Autodesk Fusion 360 part; units mm, degrees
note: some values were not read from the file. Chosen so that the rebuilt part matches the saved one: where a step ends; which bodies a step acts on; which face or edge a step refers to. Set by a fixed rule: which sketch regions a step uses.
(part 5 of 5)
  spline S19 degree 5 poles (-12.661362, 8.043004) (-12.659845, 8.039125) (-12.656809, 8.031374) (-12.652245, 8.019765) (-12.646142, 8.004321) (-12.638485, 7.985073) (-12.630798, 7.965883) (-12.623082, 7.946751) (-12.615336, 7.927676) (-12.607562, 7.90866) (-12.599758, 7.889701) (-12.591926, 7.8708) (-12.584066, 7.851958) (-12.576177, 7.833174) (-12.568261, 7.814449) (-12.560317, 7.795783) (-12.552346, 7.777176) (-12.544347, 7.758628) (-12.536322, 7.74014) (-12.52827, 7.721712) (-12.520192, 7.703343) (-12.512088, 7.685035) (-12.503958, 7.666786) (-12.495802, 7.648598) (-12.48762, 7.63047) (-12.479414, 7.612402) (-12.471182, 7.594396) (-12.462926, 7.57645) (-12.454645, 7.558566) (-12.44634, 7.540743) (-12.438011, 7.522982) (-12.429659, 7.505282) (-12.421283, 7.487644) (-12.412883, 7.470068) (-12.404461, 7.452554) (-12.396017, 7.435102) (-12.387549, 7.417713) (-12.37906, 7.400387) (-12.370549, 7.383123) (-12.362016, 7.365923) (-12.353462, 7.348786) (-12.344887, 7.331712) (-12.336292, 7.314701) (-12.327675, 7.297755) (-12.319039, 7.280872) (-12.310382, 7.264053) (-12.301706, 7.247299) (-12.293011, 7.230609) (-12.284296, 7.213983) (-12.275563, 7.197422) (-12.266811, 7.180926) (-12.258041, 7.164495) (-12.249253, 7.14813) (-12.240448, 7.13183) (-12.231625, 7.115595) (-12.222785, 7.099426) (-12.213928, 7.083323) (-12.205055, 7.067287) (-12.196166, 7.051316) (-12.187261, 7.035412) (-12.17834, 7.019575) (-12.169405, 7.003804) (-12.160454, 6.9881) (-12.151489, 6.972464) (-12.14251, 6.956895) (-12.133517, 6.941393) (-12.12451, 6.925959) (-12.11549, 6.910593) (-12.106457, 6.895295) (-12.097411, 6.880065) (-12.088353, 6.864903) (-12.079283, 6.84981) (-12.070202, 6.834786) (-12.061109, 6.81983) (-12.052006, 6.804944) (-12.042891, 6.790127) (-12.033767, 6.775379) (-12.024633, 6.7607) (-12.015489, 6.746092) (-12.006336, 6.731553) (-11.997175, 6.717085) (-11.988004, 6.702687) (-11.978826, 6.688359) (-11.96964, 6.674102) (-11.960447, 6.659916) (-11.951247, 6.6458) (-11.94204, 6.631756) (-11.932827, 6.617783) (-11.923609, 6.603882) (-11.914384, 6.590052) (-11.905155, 6.576294) (-11.895921, 6.562608) (-11.886683, 6.548995) (-11.877441, 6.535453) (-11.868195, 6.521985) (-11.858947, 6.508589) (-11.849696, 6.495266) (-11.840442, 6.482016) (-11.831187, 6.468839) (-11.82193, 6.455736) (-11.812673, 6.442706) (-11.803415, 6.42975) (-11.794156, 6.416868) (-11.784898, 6.404061) (-11.775641, 6.391327) (-11.766385, 6.378668) (-11.757131, 6.366084) (-11.747878, 6.353575) (-11.738628, 6.34114) (-11.729382, 6.328781) (-11.720138, 6.316498) (-11.710899, 6.30429) (-11.701664, 6.292157) (-11.692433, 6.280101) (-11.683208, 6.26812) (-11.673989, 6.256217) (-11.664776, 6.244389) (-11.65557, 6.232638) (-11.646372, 6.220964) (-11.637181, 6.209367) (-11.627998, 6.197847) (-11.618824, 6.186405) (-11.60966, 6.17504) (-11.600505, 6.163753) (-11.59136, 6.152544) (-11.582227, 6.141413) (-11.573105, 6.13036) (-11.563995, 6.119386) (-11.554897, 6.108491) (-11.545813, 6.097674) (-11.536742, 6.086936) (-11.527685, 6.076278) (-11.518643, 6.065699) (-11.509617, 6.0552) (-11.500606, 6.04478) (-11.491612, 6.03444) (-11.482634, 6.024181) (-11.473675, 6.014002) (-11.464734, 6.003903) (-11.455812, 5.993885) (-11.446909, 5.983948) (-11.438026, 5.974092) (-11.429165, 5.964318) (-11.420324, 5.954624) (-11.411506, 5.945013) (-11.402711, 5.935483) (-11.393939, 5.926036) (-11.385191, 5.916671) (-11.376467, 5.907388) (-11.36777, 5.898187) (-11.359098, 5.88907) (-11.350453, 5.880036) (-11.341836, 5.871084) (-11.333247, 5.862217) (-11.324687, 5.853432) (-11.316157, 5.844732) (-11.307657, 5.836116) (-11.299189, 5.827584) (-11.290753, 5.819136) (-11.282349, 5.810773) (-11.273979, 5.802494) (-11.265644, 5.794301) (-11.257344, 5.786193) (-11.249079, 5.77817) (-11.240852, 5.770233) (-11.232662, 5.762381) (-11.224511, 5.754616) (-11.2164, 5.746937) (-11.208329, 5.739344) (-11.200299, 5.731838) (-11.192311, 5.724419) (-11.184366, 5.717087) (-11.176465, 5.709842) (-11.168609, 5.702685) (-11.160799, 5.695616) (-11.153036, 5.688634) (-11.145321, 5.68174) (-11.137655, 5.674935) (-11.130039, 5.668219) (-11.122474, 5.661591) (-11.11496, 5.655052) (-11.1075, 5.648603) (-11.100094, 5.642243) (-11.092744, 5.635973) (-11.085449, 5.629792) (-11.078213, 5.623702) (-11.071035, 5.617702) (-11.063918, 5.611793) (-11.056861, 5.605975) (-11.049867, 5.600248) (-11.042937, 5.594612) (-11.036071, 5.589068) (-11.029272, 5.583616) (-11.022541, 5.578256) (-11.015879, 5.572988) (-11.009287, 5.567813) (-11.002767, 5.562731) (-10.99632, 5.557742) (-10.989948, 5.552846) (-10.983652, 5.548044) (-10.977434, 5.543336) (-10.971295, 5.538722) (-10.965238, 5.534203) (-10.959263, 5.529778) (-10.953372, 5.525448) (-10.947568, 5.521214) (-10.941851, 5.517076) (-10.936224, 5.513033) (-10.930688, 5.509087) (-10.925246, 5.505237) (-10.919899, 5.501484) (-10.914649, 5.497828) (-10.909498, 5.49427) (-10.904449, 5.49081) (-10.899504, 5.487447) (-10.894664, 5.484184) (-10.889933, 5.481019) (-10.885311, 5.477953) (-10.880803, 5.474987) (-10.87641, 5.472121) (-10.872134, 5.469356) (-10.867979, 5.466691) (-10.863948, 5.464127) (-10.860042, 5.461665) (-10.856264, 5.459305) (-10.852619, 5.457048) (-10.849109, 5.454893) (-10.845736, 5.452842) (-10.842505, 5.450894) (-10.839418, 5.449051) (-10.836479, 5.447312) (-10.833693, 5.445679) (-10.831063, 5.444152) (-10.828592, 5.442732) (-10.826285, 5.441418) (-10.824145, 5.440212) (-10.822176, 5.439114) (-10.820385, 5.438125) (-10.818777, 5.437246) (-10.817359, 5.436478) (-10.816135, 5.43582) (-10.815312, 5.435384) (-10.814783, 5.435107) (-10.81447, 5.434944) (-10.814323, 5.434869) knots -1 -1 -1 -1 -1 -1 -0.99583333 -0.99166667 -0.9875 -0.98333333 -0.97916667 -0.975 -0.97083333 -0.96666667 -0.9625 -0.95833333 -0.95416667 -0.95 -0.94583333 -0.94166667 -0.9375 -0.93333333 -0.92916667 -0.925 -0.92083333 -0.91666667 -0.9125 -0.90833333 -0.90416667 -0.9 -0.89583333 -0.89166667 -0.8875 -0.88333333 -0.87916667 -0.875 -0.87083333 -0.86666667 -0.8625 -0.85833333 -0.85416667 -0.85 -0.84583333 -0.84166667 -0.8375 -0.83333333 -0.82916667 -0.825 -0.82083333 -0.81666667 -0.8125 -0.80833333 -0.80416667 -0.8 -0.79583333 -0.79166667 -0.7875 -0.78333333 -0.77916667 -0.775 -0.77083333 -0.76666667 -0.7625 -0.75833333 -0.75416667 -0.75 -0.74583333 -0.74166667 -0.7375 -0.73333333 -0.72916667 -0.725 -0.72083333 -0.71666667 -0.7125 -0.70833333 -0.70416667 -0.7 -0.69583333 -0.69166667 -0.6875 -0.68333333 -0.67916667 -0.675 -0.67083333 -0.66666667 -0.6625 -0.65833333 -0.65416667 -0.65 -0.64583333 -0.64166667 -0.6375 -0.63333333 -0.62916667 -0.625 -0.62083333 -0.61666667 -0.6125 -0.60833333 -0.60416667 -0.6 -0.59583333 -0.59166667 -0.5875 -0.58333333 -0.57916667 -0.575 -0.57083333 -0.56666667 -0.5625 -0.55833333 -0.55416667 -0.55 -0.54583333 -0.54166667 -0.5375 -0.53333333 -0.52916667 -0.525 -0.52083333 -0.51666667 -0.5125 -0.50833333 -0.50416667 -0.5 -0.49583333 -0.49166667 -0.4875 -0.48333333 -0.47916667 -0.475 -0.47083333 -0.46666667 -0.4625 -0.45833333 -0.45416667 -0.45 -0.44583333 -0.44166667 -0.4375 -0.43333333 -0.42916667 -0.425 -0.42083333 -0.41666667 -0.4125 -0.40833333 -0.40416667 -0.4 -0.39583333 -0.39166667 -0.3875 -0.38333333 -0.37916667 -0.375 -0.37083333 -0.36666667 -0.3625 -0.35833333 -0.35416667 -0.35 -0.34583333 -0.34166667 -0.3375 -0.33333333 -0.32916667 -0.325 -0.32083333 -0.31666667 -0.3125 -0.30833333 -0.30416667 -0.3 -0.29583333 -0.29166667 -0.2875 -0.28333333 -0.27916667 -0.275 -0.27083333 -0.26666667 -0.2625 -0.25833333 -0.25416667 -0.25 -0.24583333 -0.24166667 -0.2375 -0.23333333 -0.22916667 -0.225 -0.22083333 -0.21666667 -0.2125 -0.20833333 -0.20416667 -0.2 -0.19583333 -0.19166667 -0.1875 -0.18333333 -0.17916667 -0.175 -0.17083333 -0.16666667 -0.1625 -0.15833333 -0.15416667 -0.15 -0.14583333 -0.14166667 -0.1375 -0.13333333 -0.12916667 -0.125 -0.12083333 -0.11666667 -0.1125 -0.10833333 -0.10416667 -0.1 -0.09583333 -0.09166667 -0.0875 -0.08333333 -0.07916667 -0.075 -0.07083333 -0.06666667 -0.0625 -0.05833333 -0.05416667 -0.05 -0.04583333 -0.04166667 -0.0375 -0.03333333 -0.02916667 -0.025 -0.02083333 -0.01666667 -0.0125 -0.00833333 -0.00416667 0 0 0 0 0 0
  line L38 (-10.814323, 5.434869) -> (-10.813121, 5.43425)
  line L39 (-10.813121, 5.43425) -> (-8.376657, 4.209779)
  circle A20 centre (0, 0) radius 1
  dimension "d7" = 2
  constraint concentric A0 A20
  measures "d7" diameter of A20
hole "Hole1" at (0, 0, 10) direction (0, 0, -1) diameter 2 end through all bodies 1
scale "Scale1" factor 0.86834 about (-3.736775, 14.527096, 10) bodies 1
scale "Scale2" factor 1.15 about (4.331155, 11.250245, 1.3166) bodies 1

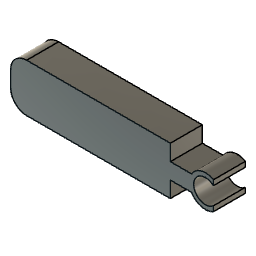
design "Pinky Finger"
Autodesk Fusion 360 part; units mm, degrees
sketch "Sketch1" plane through (0, 0, 0) normal (0, 1, 0) x (1, 0, 0)
  line L0 (0, 0) -> (50, 0)
  line L1 (0, 0) -> (0, -15)
  line L2 (0, -15) -> (50, -15)
  line L3 (50, -15) -> (50, 0)
  dimension "d1" = 50
  dimension "d2" = 15
  constraint coincident L0.start L1.start
  constraint horizontal L0
  constraint perpendicular L0 L1
  constraint perpendicular L1 L2
  constraint perpendicular L0 L3
  measures "d1" distance of L0.start L0.end
  measures "d2" distance of L0.start L1.end
extrude "Extrude1" add sketch "Sketch1" along normal blind 10
fillet "Fillet1" radius 5 2 edges at (0, 5, 15) (0, 5, 0)
sketch "Sketch2" plane through (50, 0, 0) normal (1, 0, 0) x (0, 1, 0)
  line L0 (0, 15) -> (0, 0)
  line L1 (0, 0) -> (10, 0)
  line L2 (10, 0) -> (10, 15)
  line L3 (10, 15) -> (0, 15)
  line L4 (0, 10) -> (10, 10)
  line L5 (10, 10) -> (10, 5)
  line L6 (10, 5) -> (0, 5)
  line L7 (0, 5) -> (0, 10)
  dimension "d7" = 5
  dimension "d8" = 5
  constraint horizontal L4
  constraint vertical L5
  constraint horizontal L6
  constraint vertical L7
  constraint coincident L0 L4.start
  measures "d7" distance of L4.start L6.end
  measures "d8" distance of L3 L4
extrude "Extrude2" add sketch "Sketch2" along normal blind 7.5 contours L0 L2 L4 L5 L6 L7
cylinder "CylinderPrimitive1" add diameter 10 height -10 placed x (1, 0, 0) y (0, 0, 1) z (0, -1, 0) at (60.9833, 0, 7.5)
sketch "Sketch4" plane through (0, 0, 0) normal (0, -1, 0) x (1, 0, 0)
  line L0 (56.6532, 10) -> (50, 10)
  line L1 (50, 10) -> (50, 15)
  line L2 (50, 15) -> (5, 15)
  arc A0 (5, 15) -> (0, 10) centre (5, 10) ccw
  line L3 (0, 10) -> (0, 5)
  arc A1 (0, 5) -> (5, 0) centre (5, 5) ccw
  line L4 (5, 0) -> (50, 0)
  line L5 (50, 0) -> (50, 5)
  line L6 (50, 5) -> (56.6532, 5)
  arc A2 (56.6532, 5) -> (56.6532, 10) centre (60.9833, 7.5) ccw
  circle A3 centre (60.9833, 7.5) radius 3.7
  dimension "d13" = 7.4
  constraint concentric A2 A3
  measures "d13" diameter of A3
extrude "Extrude3" cut sketch "Sketch4" against normal blind 18 contours A3
ref_plane "WorkPlane1" through (65.9833, 4.05, 7.5) normal (1, 0, 0) x (0, 0, 1)
sketch "Sketch5" plane through (65.9833, 4.05, 7.5) normal (1, 0, 0) x (0, 1, 0)
  line L0 (-6, 7) -> (8, 7)
  line L1 (8, 7) -> (8, -5)
  line L2 (8, -5) -> (-6, -5)
  line L3 (-6, -5) -> (-6, 7)
  constraint horizontal L0
  constraint vertical L1
  constraint horizontal L2
  constraint vertical L3
extrude "Extrude4" cut sketch "Sketch5" against normal blind 2.5
sketch "Sketch6" plane through (0, 0, 0) normal (0, -1, 0) x (1, 0, 0)
  line L0 (63.4833, 3.1699) -> (63.4833, 4.7724)
  arc A0 (63.4833, 10.2276) -> (63.4833, 4.7724) centre (60.9833, 7.5) ccw
  line L1 (63.4833, 10.2276) -> (63.4833, 11.8301)
  arc A1 (63.4833, 11.8301) -> (56.6532, 10) centre (60.9833, 7.5) ccw
  line L2 (56.6532, 10) -> (50, 10)
  line L3 (50, 10) -> (50, 15)
  line L4 (50, 15) -> (5, 15)
  arc A2 (5, 15) -> (0, 10) centre (5, 10) ccw
  line L5 (0, 10) -> (0, 5)
  arc A3 (0, 5) -> (5, 0) centre (5, 5) ccw
  line L6 (5, 0) -> (50, 0)
  line L7 (50, 0) -> (50, 5)
  line L8 (50, 5) -> (56.6532, 5)
  arc A4 (56.6532, 5) -> (63.4833, 3.1699) centre (60.9833, 7.5) ccw
sketch "Sketch7" plane through (0, 0, 0) normal (0, -1, 0) x (1, 0, 0)
